Autodesk Fusion 360 part; units mm, degrees
(part 2 of 2)
sketch "Sketch27" plane through (0, 16.3, 0) normal (0, -1, 0) x (1, 0, 0)
  line L0 (-32.5, 21.2) -> (-32.5, 9)
  line L1 (-32.5, 9) -> (-29.5, 9)
  line L2 (-29.5, 9) -> (-29.5, 21.2)
  line L3 (-29.5, 21.2) -> (-32.5, 21.2)
  line L4 (-32.3184, -2) -> (-2, -2)
  line L5 (-2, -2) -> (-2, 35)
  line L6 (-2, 35) -> (-32.3184, 35)
  line L7 (-32.3184, 35) -> (-32.3184, -2)
  line L8 (40.5838, -2) -> (71.4162, -2)
  line L9 (71.4162, -2) -> (71.4162, 35)
  line L10 (71.4162, 35) -> (40.5838, 35)
  line L11 (40.5838, 35) -> (40.5838, -2)
  line L12 (-2, 35) -> (40.5838, 35)
  line L13 (40.5838, 35) -> (40.5838, 24.9999)
  line L14 (40.5838, 24.9999) -> (-2, 24.9999)
  line L15 (-2, 24.9999) -> (-2, 35)
  line L16 (-32.3184, 16.5) -> (-35.3184, 16.5)
  line L17 (-35.3184, 16.5) -> (-35.3184, 11.5)
  line L18 (-35.3184, 11.5) -> (-32.3184, 11.5)
  line L19 (-32.3184, 11.5) -> (-32.3184, 16.5)
  line L20 (-32.3184, 16.5) -> (-35.5, 16.5)
  line L21 (-35.5, 16.5) -> (-35.5, 21.5)
  line L22 (-35.5, 21.5) -> (-32.3184, 21.5)
  line L23 (-32.3184, 21.5) -> (-32.3184, 16.5)
  line L24 (-17.1592, -2) -> (-22.1592, -2)
  line L25 (-17.1592, -2) -> (-12.1592, -2)
  line L26 (71.4162, 16.5) -> (74.5, 16.5)
  line L27 (74.5, 16.5) -> (74.5, 21.5)
  line L28 (74.5, 21.5) -> (71.4162, 21.5)
  line L29 (71.4162, 21.5) -> (71.4162, 16.5)
  line L30 (71.4162, 16.5) -> (74.5, 16.5)
  line L31 (74.5, 16.5) -> (74.5, 11.5)
  line L32 (74.5, 11.5) -> (71.4162, 11.5)
  line L33 (71.4162, 11.5) -> (71.4162, 16.5)
  line L34 (56, -2) -> (51, -2)
  line L35 (56, -2) -> (61, -2)
  line L36 (56, -2) -> (61, -2)
  line L37 (61, -2) -> (61, -5)
  line L38 (61, -5) -> (56, -5)
  line L39 (56, -5) -> (56, -2)
  line L40 (56, -2) -> (51, -2)
  line L41 (51, -2) -> (51, -5)
  line L42 (51, -5) -> (56, -5)
  line L43 (56, -5) -> (56, -2)
  line L44 (-17.1592, -2) -> (-12.1592, -2)
  line L45 (-12.1592, -2) -> (-12.1592, -5)
  line L46 (-12.1592, -5) -> (-17.1592, -5)
  line L47 (-17.1592, -5) -> (-17.1592, -2)
  line L48 (-17.1592, -2) -> (-22.1592, -2)
  line L49 (-22.1592, -2) -> (-22.1592, -5)
  line L50 (-22.1592, -5) -> (-17.1592, -5)
  line L51 (-17.1592, -5) -> (-17.1592, -2)
  point P0 (73.5, 0)
  dimension "d192" = 3
  dimension "d193" = 5
  dimension "d194" = 5
  dimension "d214" = 5
  dimension "d215" = 5
  constraint horizontal L4
  constraint vertical L5
  constraint horizontal L6
  constraint vertical L7
  constraint horizontal L8
  constraint vertical L9
  constraint horizontal L10
  constraint vertical L11
  constraint horizontal L12
  constraint vertical L13
  constraint horizontal L14
  constraint vertical L15
  constraint coincident L11 L13.end
  constraint horizontal L16
  constraint vertical L17
  constraint horizontal L18
  constraint vertical L19
  constraint midpoint L7 L16.start
  constraint horizontal L20
  constraint vertical L21
  constraint horizontal L22
  constraint vertical L23
  constraint horizontal L24
  constraint midpoint L4 L24.start
  constraint horizontal L25
  constraint horizontal L26
  constraint vertical L27
  constraint horizontal L28
  constraint vertical L29
  constraint midpoint L9 L26.start
  constraint horizontal L30
  constraint vertical L31
  constraint horizontal L32
  constraint vertical L33
  constraint horizontal L34
  constraint midpoint L8 L34.start
  constraint horizontal L35
  constraint horizontal L36
  constraint vertical L37
  constraint horizontal L38
  constraint vertical L39
  constraint horizontal L40
  constraint vertical L41
  constraint horizontal L42
  constraint vertical L43
  constraint horizontal L44
  constraint vertical L45
  constraint horizontal L46
  constraint vertical L47
  constraint horizontal L48
  constraint vertical L49
  constraint horizontal L50
  constraint vertical L51
  measures "d192" distance of L16.start L16.end
  measures "d193" distance of L16.start L18.end
  measures "d194" distance of L16.start L22.end
  measures "d214" distance of L24.start L25.end
  measures "d215" distance of L24.start L24.end
extrude "Extrude31" cut sketch "Sketch27" along normal blind 2.6 contours L0 L3 L7 L16 L20 L23 | L0 L3 L7 L16 L20 L21 L22 L23 | L0 L7 L16 L18 L19 L20 | L1 L2 L3 L4 L5 L6 L7 L15 L23 L24 L25 L44 L48 | L1 L2 L3 L7 L19 L23 | L8 L9 L10 L11 L13 L29 L33 L34 L35 L36 L40 | L9 L26 L27 L28 L29 L30 | L9 L26 L30 L31 L32 L33 bodies 16 17 20
extrude "Extrude32" add sketch "Sketch27" along normal blind 3 separate body contours L1 L2 L3 L4 L5 L6 L7 L15 L23 L24 L25 L44 L48 | L1 L2 L3 L7 L19 L23 | L5 L11 L12 L13 L14 L15 | L8 L9 L10 L11 L13 L29 L33 L34 L35 L36 L40 makes body 22
extrude "Extrude33" add sketch "Sketch27" along normal blind 2.7 contours L1 L2 L3 L4 L5 L6 L7 L15 L23 L24 L25 L44 L48 | L1 L2 L3 L7 L19 L23 | L8 L9 L10 L11 L13 L29 L33 L34 L35 L36 L40 bodies 22
extrude "Extrude34" cut sketch "Sketch27" along normal blind 0.3 contours L0 L3 L7 L16 L20 L23 | L0 L3 L7 L16 L20 L21 L22 L23 | L0 L7 L16 L18 L19 L20 | L9 L26 L27 L28 L29 L30 | L9 L26 L30 L31 L32 L33 bodies 22
move_body "Move62" bodies 22 to x (1, 0, 0) y (0, 1, 0) z (0, 0, 1) at (0, 0.2, 0)
sketch "Sketch28" plane through (0, 0, -7) normal (0, 0, 1) x (-1, 0, 0)
  line L0 (32.5, -35) -> (35.5, -35)
  line L1 (35.5, -35) -> (35.5, -25)
  line L2 (35.5, -25) -> (69.5, -25)
  line L3 (69.5, -25) -> (69.5, -5)
  line L4 (69.5, -5) -> (35.5, -5)
  line L5 (35.5, -5) -> (35.5, 23)
  line L6 (35.5, 23) -> (-74.5, 23)
  line L7 (-74.5, 23) -> (-74.5, 10)
  line L8 (-74.5, 10) -> (-71.5, 10)
  line L9 (-71.5, 10) -> (-71.5, 5)
  line L10 (-71.5, 5) -> (-74.5, 5)
  line L11 (-74.5, 5) -> (-74.5, -5)
  line L12 (-74.5, -5) -> (-108.5, -5)
  line L13 (-108.5, -5) -> (-108.5, -25)
  line L14 (-108.5, -25) -> (-74.5, -25)
  line L15 (-74.5, -25) -> (-74.5, -53)
  line L16 (-74.5, -53) -> (35.5, -53)
  line L17 (35.5, -53) -> (35.5, -40)
  line L18 (35.5, -40) -> (32.5, -40)
  line L19 (32.5, -40) -> (32.5, -35)
  line L20 (10, -30) -> (20, -45)
  line L21 (0, -45) -> (10, -30)
  line L22 (20, -45) -> (0, -45)
  line L23 (-50, -30) -> (-40, -45)
  line L24 (-60, -45) -> (-50, -30)
  line L25 (-40, -45) -> (-60, -45)
  line L26 (-10, -45) -> (-30, -45)
  line L27 (-20, -30) -> (-10, -45)
  line L28 (-30, -45) -> (-20, -30)
  line L29 (-10, 15) -> (-20, 0)
  line L30 (-40, 15) -> (-50, 0)
  line L31 (-20, 0) -> (-30, 15)
  line L32 (-60, 15) -> (-40, 15)
  line L33 (10, 0) -> (0, 15)
  line L34 (-50, 0) -> (-60, 15)
  line L35 (0, 15) -> (20, 15)
  line L36 (-30, 15) -> (-10, 15)
  line L37 (20, 15) -> (10, 0)
  line L38 (-15, -5) -> (-5, 10)
  line L39 (5, -5) -> (-15, -5)
  line L40 (-5, 10) -> (5, -5)
  line L41 (-45, -5) -> (-35, 10)
  line L42 (-25, -5) -> (-45, -5)
  line L43 (-35, 10) -> (-25, -5)
  line L44 (5, -25) -> (-5, -40)
  line L45 (-15, -25) -> (5, -25)
  line L46 (-5, -40) -> (-15, -25)
  line L47 (-25, -25) -> (-35, -40)
  line L48 (-45, -25) -> (-25, -25)
  line L49 (-35, -40) -> (-45, -25)
extrude "Extrude35" cut sketch "Sketch28" against normal blind 3 contours L20 L21 L22 | L23 L24 L25 | L26 L27 L28 | L29 L31 L36 | L30 L32 L34 | L33 L35 L37 | L38 L39 L40 | L41 L42 L43 | L44 L45 L46 | L47 L48 L49 bodies 16
fillet "Fillet16" radius 2 30 edges at (-20, 45, -8.5) (-10, 30, -8.5) (0, 45, -8.5) (15, 25, -8.5) (-5, 25, -8.5) (5, 40, -8.5) (10, 45, -8.5) (30, 45, -8.5) (20, 30, -8.5) (35, 40, -8.5) (45, 25, -8.5) (25, 25, -8.5) (60, 45, -8.5) (50, 30, -8.5) (40, 45, -8.5) (-20, -15, -8.5) (-10, 0, -8.5) (0, -15, -8.5) (5, -10, -8.5) (15, 5, -8.5) (-5, 5, -8.5) (20, 0, -8.5) (10, -15, -8.5) (30, -15, -8.5) (25, 5, -8.5) (45, 5, -8.5) (50, 0, -8.5) (35, -10, -8.5) (40, -15, -8.5) (60, -15, -8.5) on bodies 16
chamfer "Chamfer2" distance 8 angle 20 2 edges at (19.5, 53, -10) (19.5, -23, -10) measured on face at (-19.0108, 11.6667, -10) measured on face at (-19.0108, 11.6667, -10) on bodies 16
sketch "Sketch29" plane through (0, 16.5, 0) normal (0, 1, 0) x (-1, 0, 0)
  line L0 (-71.4162, 35) -> (-71.4162, -2)
  line L1 (-71.4162, -2) -> (-40.5838, -2)
  line L2 (-40.5838, -2) -> (-40.5838, 24.9999)
  line L3 (-40.5838, 24.9999) -> (2, 24.9999)
  line L4 (2, 24.9999) -> (2, -2)
  line L5 (2, -2) -> (32.3184, -2)
  line L6 (32.3184, -2) -> (32.3184, 35)
  line L7 (32.3184, 35) -> (-71.4162, 35)
  line L8 (32.3184, 16.5) -> (35.3184, 16.5)
  line L9 (35.3184, 16.5) -> (35.3184, 21.5)
  line L10 (35.3184, 21.5) -> (32.3184, 21.5)
  line L11 (32.3184, 21.5) -> (32.3184, 16.5)
  line L12 (32.3184, 16.5) -> (35.3184, 16.5)
  line L13 (35.3184, 16.5) -> (35.3184, 11.5)
  line L14 (35.3184, 11.5) -> (32.3184, 11.5)
  line L15 (32.3184, 11.5) -> (32.3184, 16.5)
  line L16 (-71.4162, 16.5) -> (-74.4162, 16.5)
  line L17 (-74.4162, 16.5) -> (-74.4162, 21.5)
  line L18 (-74.4162, 21.5) -> (-71.4162, 21.5)
  line L19 (-71.4162, 21.5) -> (-71.4162, 16.5)
  line L20 (-71.4162, 16.5) -> (-74.4162, 16.5)
  line L21 (-74.4162, 16.5) -> (-74.4162, 11.5)
  line L22 (-74.4162, 11.5) -> (-71.4162, 11.5)
  line L23 (-71.4162, 11.5) -> (-71.4162, 16.5)
  line L24 (-56, -2) -> (-61, -2)
  line L25 (-61, -2) -> (-61, -5)
  line L26 (-61, -5) -> (-56, -5)
  line L27 (-56, -5) -> (-56, -2)
  line L28 (-56, -2) -> (-51, -2)
  line L29 (-51, -2) -> (-51, -5)
  line L30 (-51, -5) -> (-56, -5)
  line L31 (-56, -5) -> (-56, -2)
  line L32 (17.1592, -2) -> (12.1592, -2)
  line L33 (12.1592, -2) -> (12.1592, -5)
  line L34 (12.1592, -5) -> (17.1592, -5)
  line L35 (17.1592, -5) -> (17.1592, -2)
  line L36 (17.1592, -2) -> (22.1592, -2)
  line L37 (22.1592, -2) -> (22.1592, -5)
  line L38 (22.1592, -5) -> (17.1592, -5)
  line L39 (17.1592, -5) -> (17.1592, -2)
  dimension "d216" = 3
  dimension "d217" = 3
  dimension "d218" = 5
  dimension "d219" = 3
  dimension "d220" = 3
  dimension "d221" = 5
  dimension "d222" = 5
  dimension "d223" = 5
  dimension "d224" = 5
  constraint horizontal L8
  constraint vertical L9
  constraint horizontal L10
  constraint vertical L11
  constraint midpoint L6 L8.start
  constraint horizontal L12
  constraint vertical L13
  constraint horizontal L14
  constraint vertical L15
  constraint horizontal L16
  constraint vertical L17
  constraint horizontal L18
  constraint vertical L19
  constraint midpoint L0 L16.start
  constraint horizontal L20
  constraint vertical L21
  constraint horizontal L22
  constraint vertical L23
  constraint horizontal L24
  constraint vertical L25
  constraint horizontal L26
  constraint vertical L27
  constraint midpoint L1 L24.start
  constraint horizontal L28
  constraint vertical L29
  constraint horizontal L30
  constraint vertical L31
  constraint horizontal L32
  constraint vertical L33
  constraint horizontal L34
  constraint vertical L35
  constraint midpoint L5 L32.start
  constraint horizontal L36
  constraint vertical L37
  constraint horizontal L38
  constraint vertical L39
  measures "d216" distance of L8.start L8.end
  measures "d217" distance of L8.start L8.end
  measures "d218" distance of L8.start L14.end
  measures "d219" distance of L16.start L16.end
  measures "d220" distance of L16.start L16.end
  measures "d221" distance of L16.start L22.end
  measures "d222" distance of L24.start L24.end
  measures "d223" distance of L32.start L32.end
  measures "d224" distance of L32.start L36.end
extrude "Extrude36" add sketch "Sketch29" against normal blind 2.7 contours L0 L16 L17 L18 L19 L20 | L0 L16 L20 L21 L22 L23 | L6 L8 L9 L10 L11 L12 | L6 L8 L12 L13 L14 L15 | L1 L24 L25 L26 L27 L31 | L1 L27 L28 L29 L30 L31 | L5 L35 L36 L37 L38 L39 | L5 L32 L33 L34 L35 L39 bodies 22
extrude "Extrude37" cut sketch "Sketch29" against normal blind 0.3 contours L0 L16 L17 L18 L19 L20 | L0 L16 L20 L21 L22 L23 | L6 L8 L9 L10 L11 L12 | L6 L8 L12 L13 L14 L15 | L1 L24 L25 L26 L27 L31 | L1 L27 L28 L29 L30 L31 | L5 L35 L36 L37 L38 L39 | L5 L32 L33 L34 L35 L39 bodies 22
move_body "Move63" bodies 15 19 to x (1, 0, 0) y (0, 1, 0) z (0, 0, 1) at (0, 0, -5)
move_body "Move64" bodies 16 to x (1, 0, 0) y (0, 1, 0) z (0, 0, 1) at (0, 0, 5)
move_body "Move65" bodies 2 to x (1, 0, 0) y (0, 1, 0) z (0, 0, 1) at (0, 0, -5)
sketch "Sketch30" plane through (0, 13.5, 0) normal (0, -1, 0) x (1, 0, 0)
  line L0 (-32.3184, -2) -> (-2, -2)
  line L1 (-2, -2) -> (-2, 24.9999)
  line L2 (-2, 24.9999) -> (40.5838, 24.9999)
  line L3 (40.5838, 24.9999) -> (40.5838, -2)
  line L4 (40.5838, -2) -> (71.4162, -2)
  line L5 (71.4162, -2) -> (71.4162, 35)
  line L6 (71.4162, 35) -> (-32.3184, 35)
  line L7 (-32.3184, 35) -> (-32.3184, -2)
  line L8 (-10, 20.4611) -> (50.0346, 20.4611)
  line L9 (50.0346, 20.4611) -> (50.0346, 28)
  line L10 (50.0346, 28) -> (-10, 28)
  line L11 (-10, 28) -> (-10, 20.4611)
  constraint horizontal L8
  constraint vertical L9
  constraint horizontal L10
  constraint vertical L11
extrude "Extrude38" cut sketch "Sketch30" against normal blind 3 contours L1 L2 L3 L8 L9 L10 L11 | L1 L2 L3 L8 bodies 22
sketch "Sketch31" plane through (0, 0, 0) normal (0, 0, 1) x (1, 0, 0)
  line L0 (0, 0) -> (87, 0)
  line L1 (87, 0) -> (87, 15)
  line L2 (87, 15) -> (0, 15)
  line L3 (0, 15) -> (0, 0)
  circle A0 centre (7.5284, 7.4834) radius 7.5
  circle A1 centre (79.5, 7.5) radius 7.5
  arc A2 (19.9973, 15) -> (69.9973, 15) centre (44.9973, 159.4206) ccw
  arc A3 (70, 0) -> (20, 0) centre (45, -143.2108) ccw
  line L4 (18, 12) -> (18, 3)
  line L5 (18, 3) -> (37.4872, 7.5)
  line L6 (37.4872, 7.5) -> (18, 12)
  line L7 (69, 12) -> (69, 3)
  line L8 (69, 3) -> (49.5128, 7.5)
  line L9 (49.5128, 7.5) -> (69, 12)
  circle A4 centre (7.5284, 7.4834) radius 3.75
  circle A5 centre (79.5, 7.5) radius 3.75
  line L10 (10.0045, 10.2997) -> (10.0045, 4.5997)
  line L11 (77.0229, 10.3154) -> (77.0229, 4.6154)
  line L12 (10.0045, 10.2997) -> (20, 9.5)
  line L13 (10.0045, 4.5997) -> (20, 5.5)
  line L14 (20, 5.5) -> (20, 9.5)
  line L15 (10.0045, 10.2997) -> (20, 9.5)
  line L16 (20, 5.5) -> (20, 9.5)
  line L17 (10.0045, 4.5997) -> (20, 5.5)
  line L18 (77.0229, 10.3154) -> (67.0505, 9.5739)
  line L19 (77.0229, 4.6154) -> (67.0505, 5.357)
  dimension "d235" = 87
  dimension "d236" = 15
  dimension "d237" = 15
  dimension "d238" = 15
  dimension "d239" = 20
  dimension "d240" = 7.5
  dimension "d241" = 7.5
  dimension "d243" = 5.7
  dimension "d244" = 5.7
  dimension "d248" = 5.7
  dimension "d249" = 10
  dimension "d250" = 10
  constraint horizontal L0
  constraint vertical L1
  constraint horizontal L2
  constraint vertical L3
  constraint coincident L0.start L3.end
  constraint coincident L2 A2.start
  constraint coincident L0 A3.start
  constraint coincident L0 A3.end
  constraint perpendicular L2 L4
  constraint perpendicular L2 L7
  constraint parallel L6 L8
  constraint concentric A0 A4
  constraint concentric A1 A5
  constraint vertical L10
  constraint coincident A4 L10.start
  constraint vertical L11
  constraint coincident A5 L11.start
  constraint parallel L4 L14
  measures "d235" distance of L0.start L0.end
  measures "d236" distance of L0.start L2.end
  measures "d237" diameter of A0
  measures "d238" diameter of A1
  measures "d239" distance of L4.end L5.end
  measures "d240" diameter of A4
  measures "d241" diameter of A5
  measures "d243" distance of L10.start L10.end
  measures "d244" distance of L11.start L11.end
  measures "d248" distance of L10.start L10.end
  measures "d249" distance of L11.start L18.end
  measures "d250" distance of L11.end L19.end
extrude "Extrude39" add sketch "Sketch31" along normal blind 4 separate body contours L0 L2 L3 A0 A1 A2 A3 L4 L5 L6 L7 L8 L9 L12 L13 L15 L17 L18 L19 | L0 A0 A4 L10 L12 L13 L15 L17 | A1 A5 L11 L18 L19 | A0 A4 L10 L12 L13 L15 L17 | A0 L4 L12 L13 L15 L17 | A1 L7 L18 L19 | A1 A5 L11 L18 L19 makes body 23
fillet "Fillet19" radius 7.5 2 edges at (0, 0, 2) (0, 15, 2) on bodies 23
fillet "Fillet20" radius 1 6 edges at (18, 12, 2) (18, 3, 2) (37.4872, 7.5, 2) (49.5128, 7.5, 2) (69, 12, 2) (69, 3, 2) on bodies 23
extrude "Extrude40" cut sketch "Sketch31" along normal blind 1.5 contours A0 A4 L10 L12 L13 L15 L17 | A0 L4 L12 L13 L15 L17 | A1 L7 L18 L19 | A1 A5 L11 L18 L19 picked at (73.3239, 6.6204) bodies 23
sketch "Sketch32" plane through (0, 0, 0) normal (0, 0, 1) x (1, 0, 0)
  line L0 (0, 0) -> (87, 0)
  line L1 (87, 0) -> (87, 16)
  line L2 (87, 16) -> (0, 16)
  line L3 (0, 16) -> (0, 0)
  line L4 (59.2, 1.8) -> (82, 1.8)
  line L5 (82, 1.8) -> (82, 14)
  line L6 (82, 14) -> (59.2, 14)
  line L7 (59.2, 14) -> (59.2, 1.8)
  circle A0 centre (8, 8) radius 8
  arc A1 (15.2121, 16) -> (54.048, 16) centre (34.6301, 203.9599) ccw
  spline S0 degree 5 poles (12, 0) (12.1401, -0.0365) (12.4272, -0.0997) (12.8778, -0.165) (13.5189, -0.1929) (14.3838, -0.1277) (15.3019, 0.0413) (16.2507, 0.3218) (17.1963, 0.7244) (18.1048, 1.2562) (18.9521, 1.9156) (19.7333, 2.6867) (20.4743, 3.5335) (21.2212, 4.4066) (22.0288, 5.2522) (22.9497, 6.0202) (24.0232, 6.672) (25.2634, 7.1892) (26.6641, 7.5694) (28.2034, 7.8219) (29.848, 7.9637) (31.5578, 8.0152) (33.2903, 7.9967) (35.0053, 7.9233) (36.6672, 7.8048) (38.246, 7.6469) (39.7197, 7.4515) (41.0754, 7.2176) (42.3112, 6.9418) (43.438, 6.6194) (44.4803, 6.2446) (45.4687, 5.813) (46.4346, 5.3231) (47.4042, 4.7782) (48.3917, 4.1882) (49.3972, 3.5703) (50.412, 2.945) (51.4223, 2.3336) (52.4129, 1.7556) (53.3722, 1.2255) (54.2934, 0.7515) (54.9972, 0.4203) (55.506, 0.1994) (55.8367, 0.0644) (56, 0) knots 0 0 0 0 0 0 0.025 0.05 0.075 0.1 0.125 0.15 0.175 0.2 0.225 0.25 0.275 0.3 0.325 0.35 0.375 0.4 0.425 0.45 0.475 0.5 0.525 0.55 0.575 0.6 0.625 0.65 0.675 0.7 0.725 0.75 0.775 0.8 0.825 0.85 0.875 0.9 0.925 0.95 0.975 1 1 1 1 1 1
  circle A2 centre (8, 8) radius 5
  circle A3 centre (8, 8) radius 3
  spline S1 degree 5 poles (16, 13) (17.5333, 13) (20.6, 13) (25.2, 13) (31.3333, 13) (39, 13) (45.1333, 13) (49.7333, 13) (52.8, 13) (54.3333, 13) knots 0 0 0 0 0 0 0.2 0.4 0.6 0.8 1 1 1 1 1 1
  line L8 (54.3333, 13) -> (54.3333, 6)
  spline S2 degree 5 poles (54.3333, 6) (53.9336, 6.2334) (53.1459, 6.6841) (51.9995, 7.3113) (50.5412, 8.0499) (48.8338, 8.8106) (47.2357, 9.4112) (45.733, 9.8584) (44.3023, 10.1641) (42.9063, 10.348) (41.4967, 10.4371) (40.0253, 10.4612) (38.4529, 10.4499) (36.7592, 10.4293) (34.9523, 10.4182) (33.0609, 10.4258) (31.1267, 10.4488) (29.1967, 10.4681) (27.3159, 10.4473) (25.5184, 10.3263) (23.8251, 10.0302) (22.2488, 9.4939) (20.7982, 8.6842) (19.481, 7.6203) (18.3086, 6.4023) (17.298, 5.2129) (16.4675, 4.2707) (15.8346, 3.7968) (15.4133, 3.9725) (15.2112, 4.9112) (15.232, 6.6777) (15.4276, 8.7756) (15.6748, 10.7372) (15.8842, 12.217) (16, 13) knots 0 0 0 0 0 0 0.033333 0.066667 0.1 0.133333 0.166667 0.2 0.233333 0.266667 0.3 0.333333 0.366667 0.4 0.433333 0.466667 0.5 0.533333 0.566667 0.6 0.633333 0.666667 0.7 0.733333 0.766667 0.8 0.833333 0.866667 0.9 0.933333 0.966667 1 1 1 1 1 1
  circle A4 centre (84.9678, 7.9) radius 0.9006
  circle A5 centre (56.2856, 7.9) radius 0.9442
  line L9 (25, 10) -> (30, 10)
  line L10 (30, 10) -> (30, 14)
  line L11 (30, 14) -> (25, 14)
  line L12 (25, 14) -> (25, 10)
  line L13 (39, 14) -> (44, 14)
  line L14 (44, 14) -> (44, 10)
  line L15 (44, 10) -> (39, 10)
  line L16 (39, 10) -> (39, 14)
  point P0 (15, 0)
  point P1 (19, 2)
  point P2 (23, 6)
  point P3 (32, 8)
  point P4 (42, 7)
  point P5 (47, 5)
  point P6 (52, 2)
  point P7 (45, 10)
  point P8 (38.4099, 10.4474)
  point P9 (28.1821, 10.4474)
  point P10 (20, 8)
  point P11 (16, 4)
  dimension "d259" = 87
  dimension "d260" = 16
  dimension "d261" = 22.8
  dimension "d262" = 12.2
  constraint horizontal L0
  constraint vertical L1
  constraint horizontal L2
  constraint vertical L3
  constraint coincident L0.start L3.end
  constraint horizontal L4
  constraint vertical L5
  constraint horizontal L6
  constraint vertical L7
  constraint coincident L2 A1.start
  constraint coincident L2 A1.end
  constraint coincident L0 S0.start
  constraint coincident L0 P0
  constraint coincident L0 S0.end
  constraint concentric A0 A2
  constraint concentric A0 A3
  constraint perpendicular L2 L8
  constraint horizontal L9
  constraint vertical L10
  constraint horizontal L11
  constraint vertical L12
  constraint horizontal L13
  constraint vertical L14
  constraint horizontal L15
  constraint vertical L16
  measures "d259" distance of L0.start L0.end
  measures "d260" distance of L0.start L2.end
  measures "d261" distance of L4.start L4.end
  measures "d262" distance of L4.start L6.end
extrude "Extrude41" add sketch "Sketch32" along normal blind 4 separate body contours L0 L1 L2 A0 A1 S0 S1 L8 S2 L9 L10 L11 L12 L13 L14 L15 L16 | A0 S2 | S2 L9 L10 L12 | S1 L10 L11 L12 | S2 L14 L15 L16 | S1 L13 L14 L16 | A2 picked at (14.6225, 8.6595) makes body 24
fillet "Fillet21" radius 5.5 2 edges at (87, 16, 2) (87, 0, 2) on bodies 24
fillet "Fillet22" radius 1.5 3 edges at (16, 13, 2) (54.3333, 13, 2) (54.3333, 6, 2) on bodies 24
extrude "Extrude42" cut sketch "Sketch32" along normal blind 5 contours A2 bodies 24
extrude "Extrude43" add sketch "Sketch32" along normal blind 3 contours A2 bodies 24
extrude "Extrude44" cut sketch "Sketch32" along normal blind 1 contours A2 bodies 24
extrude "Extrude45" add sketch "Sketch32" along normal blind 3 contours S1 S2 L10 L12 | S1 S2 L14 L16 bodies 24
extrude "Extrude46" cut sketch "Sketch32" along normal blind 1 contours S1 S2 L10 L12 | S1 S2 L14 L16 bodies 24
move_body "Move66" bodies 23 to x (0, 0, -1) y (-1, 0, 0) z (0, 1, 0) at (104.2673, 62, 22.756)
hidden bodies 2 1 4 5 6 8 7 10 9 11 12 13 19 20 21
named bodies: "servo1.1", "holder", "servo1", "servo2.1", "servo1 (1)", "servo1 (2)", "servo3.1", "servo4.1", "servo1 (3)", "servo2", "servo3", "servo4", "servo2.2", "servo1.2", "servo4.2", "servo3.2", "kreplenie_pov 1", "kreplenie_pov 2", "kreplenie_pov 1 (1)", "kreplenie_pov 3", "kreplenie_pov 1 (2)", "kreplenie_pov 4", "zad", "niz", "seredina_zad", "soedinenie1", "pered", "seredina_pered", "soedinenie", "soedinenie2", "seredina"
